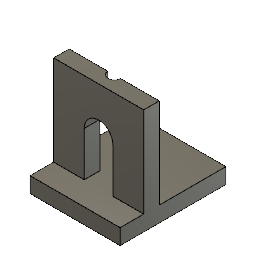
Soporte Potenciometro v5 (Autodesk Fusion 360 design; units mm, degrees)
Autodesk Fusion 360 part; units mm, degrees
note: some values were not read from the file. Set by a fixed rule: which sketch regions a step uses.
sketch "Sketch1" plane through (0, 0, 0) normal (0, 1, 0) x (1, 0, 0)
  line L0 (0, 0) -> (23, 0)
  line L1 (23, 0) -> (23, 27)
  line L2 (23, 27) -> (0, 27)
  line L3 (0, 27) -> (0, 0)
  line L4 (11.5, 0) -> (11.5, 27)
  line L5 (11.5, 0) -> (11.5, 6)
  line L6 (23, 6) -> (0, 6)
  line L7 (11.5, 6) -> (11.5, 10)
  line L8 (0, 6) -> (23, 6)
  line L9 (23, 6) -> (23, 10)
  line L10 (23, 10) -> (0, 10)
  line L11 (0, 10) -> (0, 6)
  dimension "d1" = 23
  dimension "d2" = 27
  dimension "d3" = 6
  dimension "d4" = 4
  constraint horizontal L0
  constraint vertical L1
  constraint horizontal L2
  constraint vertical L3
  constraint coincident L0.start L3.end
  constraint midpoint L0 L4.start
  constraint midpoint L2 L4.end
  constraint perpendicular L0 L5
  constraint coincident L1 L6.start
  constraint coincident L3 L6.end
  constraint perpendicular L3 L6
  constraint perpendicular L6 L7
  constraint horizontal L8
  constraint vertical L9
  constraint horizontal L10
  constraint vertical L11
  constraint coincident L1 L9.end
  measures "d1" distance of L0.start L0.end
  measures "d2" distance of L0.start L2.end
  measures "d3" distance of L4.start L5.end
  measures "d4" distance of L5.end L7.end
extrude "Extrude1" add sketch "Sketch1" along normal blind 4
sketch "Sketch2" plane through (0, 4, 0) normal (0, 1, 0) x (-1, 0, 0)
  line L0 (0, -27) -> (0, 0)
  line L1 (0, 0) -> (-23, 0)
  line L2 (-23, 0) -> (-23, -27)
  line L3 (-23, -27) -> (0, -27)
  line L4 (-11.5, 0) -> (-11.5, -6)
  line L5 (-23, -6) -> (0, -6)
  line L6 (0, -6) -> (0, -10)
  line L7 (0, -6) -> (-23, -6)
  line L8 (-23, -10) -> (-23, -6)
  line L9 (-23, -10) -> (0, -10)
  dimension "d7" = 6
  dimension "d8" = 4
  constraint midpoint L1 L4.start
  constraint perpendicular L1 L4
  constraint coincident L2 L5.start
  constraint coincident L0 L5.end
  constraint perpendicular L0 L5
  constraint perpendicular L5 L6
  constraint coincident L2 L8.start
  constraint perpendicular L0 L9
  measures "d7" distance of L4.start L4.end
  measures "d8" distance of L5.end L6.end
extrude "Extrude2" add sketch "Sketch2" along normal blind 23 contours L0 L2 L5 L6 L7 L8 L9
sketch "Sketch3" plane through (0, 0, -6) normal (0, 0, 1) x (1, 0, 0)
  line L0 (0, 4) -> (23, 4)
  line L1 (23, 4) -> (23, 27)
  line L2 (23, 27) -> (0, 27)
  line L3 (0, 27) -> (0, 4)
  line L4 (11.5, 0) -> (11.5, 19)
  circle A0 centre (11.5003, 15.35) radius 3.65
  line L5 (15.1503, 15.35) -> (15.1503, 4)
  line L6 (7.8503, 4) -> (7.8503, 15.35)
  dimension "d11" = 19
  dimension "d12" = 7.3
  constraint perpendicular L0 L4
  constraint coincident L4.end A0
  constraint coincident A0 L5.start
  constraint tangent A0 L5
  constraint coincident L0 L5.end
  constraint perpendicular L0 L5
  constraint coincident L0 L6.start
  constraint coincident A0 L6.end
  constraint tangent A0 L6
  constraint perpendicular L0 L6
  measures "d11" distance of L4.start L4.end
  measures "d12" diameter of A0
extrude "Extrude5" cut sketch "Sketch3" against normal blind 4 contours L0 L4 A0 L6 | L0 L4 A0 L5 | L4 A0 | L4 A0
sketch "Sketch4" plane through (0, 27, 0) normal (0, 1, 0) x (-1, 0, 0)
  line L0 (0, -6) -> (-23, -6)
  line L1 (-23, -6) -> (-23, -10)
  line L2 (-23, -10) -> (0, -10)
  line L3 (0, -10) -> (0, -6)
  circle A0 centre (-11.5, -10) radius 1.6
  dimension "d15" = 3.2
  constraint midpoint L2 A0.centre
  measures "d15" diameter of A0
extrude "Extrude4" cut sketch "Sketch4" against normal blind 9 contours L2 A0 picked at (-11.109, -9.6372)
